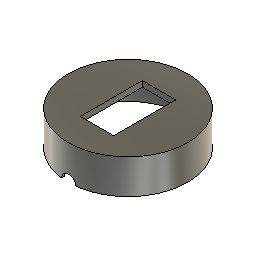
base_bottom_part_Asheeyana_Ahmed (Autodesk Fusion 360 design; units mm, degrees)
Autodesk Fusion 360 part; units mm, degrees
sketch "Sketch1" plane through (0, 0, 0) normal (0, 0, 1) x (1, 0, 0)
  line L0 (34.925, 31.75) -> (-34.925, 31.75)
  line L1 (-34.925, 31.75) -> (-34.925, -31.75)
  line L2 (-34.925, -31.75) -> (34.925, -31.75)
  line L3 (34.925, -31.75) -> (34.925, 31.75)
  line L4 (34.925, 31.75) -> (-34.925, -31.75) construction
  line L5 (-34.925, 31.75) -> (34.925, -31.75) construction
  circle A0 centre (0, 0) radius 62.5
  dimension "d1" = 69.85
  dimension "d2" = 63.5
  dimension "d3" = 125
  constraint horizontal L0
  constraint perpendicular L0 L1
  constraint parallel L0 L2
  constraint parallel L1 L3
  constraint coincident L4 A0.centre
  constraint coincident L5 A0.centre
  constraint coincident A0.centre origin
  measures "d1" distance of L1.end L2.end
  measures "d2" distance of L0.end L1.end
  measures "d3" diameter of A0
extrude "Extrude1" add sketch "Sketch1" along normal blind 31.75 contours L0 L1 L2 L3 | A0
extrude "Extrude2" cut sketch "Sketch1" along normal blind 20.32 contours L0 L1 L2 L3
sketch "Sketch3" plane through (0, 0, 31.75) normal (0, 0, 1) x (-1, 0, 0)
  circle A0 centre (0, 0) radius 62.5
  line L0 (-17.5, 32.5) -> (17.5, 32.5)
  line L1 (17.5, 32.5) -> (17.5, -32.5)
  line L2 (17.5, -32.5) -> (-17.5, -32.5)
  line L3 (-17.5, -32.5) -> (-17.5, 32.5)
  line L4 (-17.5, 32.5) -> (17.5, -32.5) construction
  line L5 (17.5, 32.5) -> (-17.5, -32.5) construction
  circle A1 centre (0, 0) radius 35
  dimension "d23" = 35
  dimension "d24" = 65
  dimension "d25" = 70
  constraint horizontal L0
  constraint perpendicular L0 L1
  constraint parallel L0 L2
  constraint parallel L1 L3
  constraint coincident L4 A0.centre
  constraint coincident L5 A0.centre
  constraint coincident A0.centre A1.centre
  measures "d23" distance of L1.end L2.end
  measures "d24" distance of L0.end L1.end
  measures "d25" diameter of A1
extrude "Extrude12" cut sketch "Sketch1" along normal blind 60 contours L0 L1 L2 L3 | A0
extrude "Extrude5" add sketch "Sketch3" along normal blind 36 contours A0 | L0 A1 | L3 A1 | L1 A1 | L2 A1
shell "Shell4" thickness 3 removed faces 1 at (32.5, 0, 31.75)
extrude "Extrude13" cut 1 faces at (19.5, 10.1036, 31.75) along direction (0, 0, 1) blind 30
ref_plane "WorkPlane1" through (0, -65, 0) normal (0, 1, 0) x (0, 0, 1)
sketch "Sketch7" plane through (0, -65, 0) normal (0, 1, 0) x (1, 0, 0)
  circle A0 centre (0.0696, -31.6703) radius 7.5
  dimension "d54" = 15
  measures "d54" diameter of A0
extrude "Extrude14" cut sketch "Sketch7" along normal blind 230
